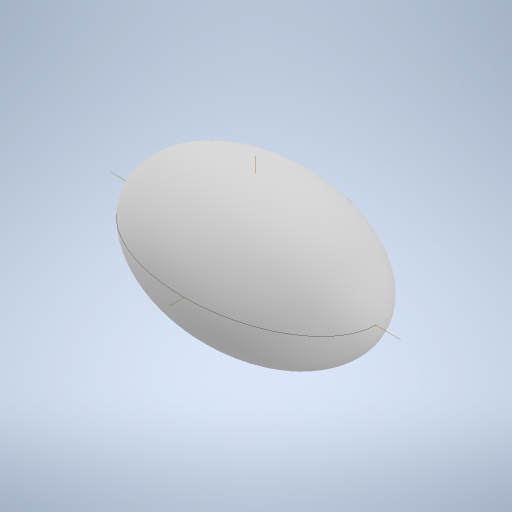
# Autodesk Inventor part: Ellipsoid
Saved by Autodesk Inventor 2023.1 (Build 271208000, 208)
## iProperties
Created: 2023-01-19
Part Number: Ellipsoid
Material: Generisch
Document SubType Name: Modeling
Designer: mehan
Density: 1 g/cm^3
Appearance: Vorgabe
Author: mehan
Autodesk Inventor part; units mm, degrees
ref_plane "YZ Plane" through (0, 0, 0) normal (1, 0, 0) x (0, 1, 0)
ref_plane "XZ Plane" through (0, 0, 0) normal (0, 1, 0) x (-1, 0, 0)
ref_plane "XY Plane" through (0, 0, 0) normal (0, 0, 1) x (1, 0, 0)
sketch "Skizze1" plane through (0, 0, 0) normal (0, 1, 0) x (-1, 0, 0)
  ellipse E0 centre (0, 0) end of major axis (-75, 0) minor radius 45 (75, 0) -> (-75, 0) ccw
  line L0 (-75, 0) -> (75, 0)
  dimension "d10" = 90
  constraints: 2 end point, 1 horizontal, 4 other
revolve "Umdrehung2" add sketch "Skizze1" angle 360 about axis through (75, 0, 0) along (-1, 0, 0)
